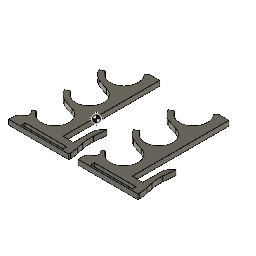
lokaverkefni_lappir_final (Autodesk Fusion 360 design; units mm, degrees)
Autodesk Fusion 360 part; units mm, degrees
sketch "Sketch1" plane through (0, 0, 0) normal (0, 0, 1) x (1, 0, 0)
  line L0 (34.445, 101.1531) -> (37.0871, 100)
  arc A0 (15.1934, 27.8106) -> (21.2794, 18.3659) centre (60, 50) ccw
  arc A1 (24.2675, 32.0225) -> (70.2683, 88.6596) centre (60, 50) ccw
  arc A2 (34.445, 101.1531) -> (70.2683, 88.6596) centre (134.445, 330.2819) ccw
  line L1 (50.2426, 114.2585) -> (49.0508, 111.5277)
  arc A3 (10.6816, 125.6547) -> (38.9202, 99.2) centre (60, 150) ccw
  arc A4 (24.2808, 131.9962) -> (70.2683, 188.6596) centre (60, 150) ccw
  arc A5 (36.6337, 200.2103) -> (70.2683, 188.6596) centre (134.445, 430.2819) ccw
  line L2 (88.2384, 278.3301) -> (95.3094, 285.4012)
  line L3 (60, 250) -> (120.6972, 250) construction
  arc A6 (24.2808, 231.9962) -> (88.2384, 278.3301) centre (60, 250) ccw
  arc A7 (10.6816, 225.6547) -> (36.6337, 200.2103) centre (60, 250) ccw
  line L4 (22.7381, 243.2768) -> (36.5507, 243.2768) construction
  line L5 (15.1934, 27.8106) -> (24.2675, 32.0225)
  line L6 (10.6816, 125.6547) -> (24.2808, 131.9962)
  line L7 (10.6816, 225.6547) -> (22.7381, 231.2768)
  line L8 (22.7381, 231.2768) -> (24.2808, 231.9962)
  line L9 (19.271, 3.8476) -> (10.7481, -2.1202)
  line L10 (22.2568, 7.1468) -> (4.2808, 7.1468) construction
  line L11 (8.9321, -3.3918) -> (9.2648, -3.3918) construction
  line L12 (132.7141, 248.2311) -> (132.6969, 250.0757)
  line L13 (7.8236, -5.3117) -> (6.5405, -7.5341)
  line L14 (8.9321, -3.3918) -> (9.2648, -3.3918) construction
  line L15 (168.0417, 91.0528) -> (216.7808, 91.0528) construction
  arc A8 (19.271, 3.8476) -> (21.2794, 18.3659) centre (13.5353, 12.0391) ccw
  arc A9 (10.7481, -2.1202) -> (7.8236, -5.3117) centre (16.4838, -10.3117) ccw
  arc A10 (6.5405, -7.5341) -> (5.2029, -12.3246) centre (15.2007, -12.5341) ccw
  line L16 (179.1661, -24.8465) -> (179.1661, -23.5067)
  line L17 (5.2029, -12.3246) -> (4.9961, -22.1946)
  line L18 (17.1671, -29.5067) -> (179.1661, -29.5067)
  line L19 (179.1661, -29.5067) -> (179.1661, -23.5067)
  line L20 (98.1666, -29.5067) -> (98.1666, -24.5067)
  line L21 (98.1666, -24.5067) -> (38.1666, -24.5067)
  line L22 (98.1666, -24.5067) -> (158.1666, -24.5067)
  line L23 (126.3128, 6.8881) -> (126.3128, 286.8881)
  line L24 (95.3094, 285.4012) -> (96.7963, 286.8881)
  line L25 (126.3128, 286.8881) -> (96.7963, 286.8881)
  line L26 (126.3128, 6.8881) -> (156.3128, 6.8881)
  line L27 (156.3128, 6.8881) -> (156.3128, 60.2423)
  line L28 (4.9412, -27.4331) -> (4.9412, -29.5067)
  line L29 (17.1671, -29.5067) -> (4.9412, -29.5067)
  arc A11 (4.9961, -22.1946) -> (4.9412, -27.4331) centre (254.9412, -27.4331) ccw
  line L30 (163.3423, 77.2129) -> (173.2834, 87.154)
  line L31 (156.3128, 70.1834) -> (180.3128, 70.1834) construction
  line L32 (173.2834, 87.154) -> (170.0976, 50.7401)
  line L33 (173.2834, 87.154) -> (226.6167, 87.154) construction
  line L34 (179.1661, -24.8465) -> (179.1661, -24.8301)
  line L35 (176.5391, -1.1543) -> (172.3137, 17.6514)
  arc A12 (170.0976, 50.7401) -> (172.3137, 17.6514) centre (277.6866, 41.3272) ccw
  arc A13 (179.1661, -24.8301) -> (176.5391, -1.1543) centre (71.1661, -24.8301) ccw
  arc A14 (163.3423, 77.2129) -> (156.3128, 60.2423) centre (180.3128, 60.2423) ccw
  line L36 (38.1666, -24.5067) -> (38.1666, -14.5067)
  line L37 (38.1666, -14.5067) -> (158.1666, -14.5067)
  line L38 (158.1666, -14.5067) -> (158.1666, -24.5067)
  point P0 (6.4321, -7.7219)
  point P1 (157.8394, 81.2593)
  point P2 (162.8123, 31.2811)
  point P3 (156.3128, 81.8881)
  point P4 (168.6351, 34.0236)
  point P5 (179.1661, -12.8465)
  dimension "d10" = 80
  dimension "d11" = 100
  dimension "d12" = 80
  dimension "d13" = 100
  dimension "d16" = 100
  dimension "d19" = 80
  dimension "d21" = 250
  dimension "d22" = 250
  dimension "d23" = 45
  dimension "d24" = 50
  dimension "d33" = 12
  dimension "d43" = 12
  dimension "d44" = 35
  dimension "d65" = 120
  dimension "d66" = 5
  dimension "d71" = 14.1421
  dimension "d74" = 60
  dimension "d79" = 10
  dimension "d80" = 10
  dimension "d81" = 10
  dimension "d92" = 6
  dimension "d93" = 5
  dimension "d94" = 60
  dimension "d95" = 60
  dimension "d230" = 280
  dimension "d233" = 30
  dimension "d234" = 75
  dimension "d238" = 250
  dimension "d239" = 24
  dimension "d240" = 45
  dimension "d241" = 95
  dimension "d242" = 53.3333
  dimension "d243" = 12
  dimension "d244" = 108
  dimension "d245" = 24
  dimension "d246" = 10
  dimension "d247" = 90
  dimension "d248" = 120
  dimension "d249" = 10
  constraint concentric A0 A1
  constraint concentric A6 A7
  constraint coincident L0.end A3
  constraint coincident L0 A3.end
  constraint tangent L0 A2
  constraint tangent A1 A2
  constraint coincident L1.end A4
  constraint tangent A4 A5
  constraint horizontal L3
  constraint coincident L3.start A6.centre
  constraint horizontal L4
  constraint horizontal L10
  constraint horizontal L11
  constraint horizontal L14
  constraint horizontal L15
  constraint tangent A0 A8
  constraint tangent L9 A8
  constraint coincident L11.start L9
  constraint coincident L11.start L13
  constraint tangent L9 A9
  constraint tangent L13 A9
  constraint coincident P0 L13
  constraint tangent L13 A10
  constraint coincident A9 L11.end
  constraint coincident A8 L10.start
  constraint vertical L16
  constraint tangent A10 L17
  constraint horizontal L18
  constraint vertical L19
  constraint midpoint L18 L20.start
  constraint perpendicular L18 L20
  constraint perpendicular L20 L21
  constraint perpendicular L20 L22
  constraint vertical L23
  constraint parallel L2 L24
  constraint horizontal L25
  constraint perpendicular L23 L26
  constraint perpendicular L26 L27
  constraint coincident P3 L27
  constraint vertical L28
  constraint horizontal L29
  constraint tangent L28 A11
  constraint tangent L17 A11
  constraint horizontal L31
  constraint horizontal L33
  constraint parallel L16 L34
  constraint coincident P4 L32
  constraint coincident P4 L35
  constraint tangent L32 A12
  constraint tangent L35 A12
  constraint coincident P5 L35
  constraint coincident P5 L34
  constraint tangent L35 A13
  constraint tangent L34 A13
  constraint equal A12 A13
  constraint coincident L31.start L30
  constraint coincident L27 L31.start
  constraint tangent L30 A14
  constraint tangent L27 A14
  constraint perpendicular L21 L36
  constraint perpendicular L37 L38
  measures "d10" diameter of A1
  measures "d11" distance of A0.centre A3.centre
  measures "d12" diameter of A4
  measures "d13" distance of A3.centre L3.start
  measures "d16" diameter of A0
  measures "d19" diameter of A6
  measures "d21" radius of A2
  measures "d22" radius of A5
  measures "d23" angle of L2 L3
  measures "d24" distance of L3.start L2.end
  measures "d33" distance of L3.end L12.end
  measures "d43" distance of L4.start L7.end
  measures "d44" angle of L9 L10
  measures "d65" angle of L13 L14
  measures "d66" distance of L11.start P0
  measures "d71" distance of P1 L15.start
  measures "d74" distance of L15.start P2
  measures "d79" radius of A8
  measures "d80" radius of A9
  measures "d81" radius of A10
  measures "d92" distance of L16.end L18.end
  measures "d93" distance of L20.start L20.end
  measures "d94" distance of L20.end L21.end
  measures "d95" distance of L20.end L22.end
  measures "d230" distance of L23.start L23.end
  measures "d233" distance of L23.start L26.end
  measures "d234" distance of L26.end P3
  measures "d238" radius of A11
  measures "d239" distance of L31.start L30.end
  measures "d240" angle of L30 L31
  measures "d241" angle of L32 L33
  measures "d242" distance of L30.end P4
  measures "d243" distance of L16.start P5
  measures "d244" radius of A12
  measures "d245" radius of A14
  measures "d246" distance of L21.end L36.end
  measures "d247" angle of L36 L37
  measures "d248" distance of L36.end L37.end
  measures "d249" distance of L37.end L22.end
extrude "Extrude1" add sketch "Sketch1" along normal blind 12 contours A0 A1 A2 A3 A4 A5 L2 A6 A7 L5 L6 L7 L8 L9 L13 A8 A9 A10 L16 L17 L18 L19 L23 L24 L25 L26 L27 L28 L29 A11 L30 L32 L34 L35 A12 A13 A14 makes body 1
copy_body "CopyPasteBodies1" bodies 1 makes body 2
move_body "Move1" bodies 2 to x (1, 0, 0) y (0, 1, 0) z (0, 0, 1) at (0, 0, 200)
ref_plane "WorkPlane1" through (98.1666, -24.5067, 6) normal (0, 1, 0) x (-1, 0, 0)
sketch "Sketch2" plane through (0, -24.5067, 0) normal (0, 1, 0) x (1, 0, 0)
  line L0 (0, 0) -> (120, 0)
  line L1 (120, 0) -> (120, -174)
  line L2 (120, -174) -> (0, -174)
  line L3 (0, -174) -> (0, 0)
  dimension "d103" = 120
  dimension "d104" = 174
  constraint horizontal L0
  constraint vertical L1
  constraint horizontal L2
  constraint vertical L3
  constraint coincident L0.start L3.end
  measures "d103" distance of L0.start L0.end
  measures "d104" distance of L0.start L2.end
extrude "Extrude2" add sketch "Sketch2" along normal blind 10 separate body makes body 3
sketch "Sketch3" plane through (0, -14.5067, 0) normal (0, 1, 0) x (-1, 0, 0)
  line L0 (0, 174) -> (-120, 174)
  line L1 (-120, 174) -> (-120, 0)
  line L2 (-120, 0) -> (0, 0)
  line L3 (0, 0) -> (0, 174)
  line L4 (-120, 0) -> (0, 0)
  line L5 (0, 0) -> (0, 17)
  line L6 (0, 17) -> (-120, 17)
  line L7 (-120, 17) -> (-120, 0)
  line L8 (0, 174) -> (-120, 174)
  line L9 (-120, 174) -> (-120, 157)
  line L10 (-120, 157) -> (0, 157)
  line L11 (0, 157) -> (0, 174)
  dimension "d107" = 120
  dimension "d108" = 17
  dimension "d109" = 120
  dimension "d110" = 17
  constraint horizontal L4
  constraint vertical L5
  constraint horizontal L6
  constraint vertical L7
  constraint coincident L1.end L2.start
  constraint horizontal L8
  constraint vertical L9
  constraint horizontal L10
  constraint vertical L11
  constraint coincident L0.start L3.end
  measures "d107" distance of L1.end L2.end
  measures "d108" distance of L1.end L6.end
  measures "d109" distance of L0.start L0.end
  measures "d110" distance of L0.start L10.end
extrude "Extrude3" cut sketch "Sketch3" against normal blind 4 contours L0 L1 L3 L8 L9 L10 L11 | L1 L2 L3 L4 L5 L6 L7 bodies 3
fillet "Fillet1" radius 6 2 edges at (120, -21.5067, 0) (0, -21.5067, 0) on bodies 3
fillet "Fillet2" radius 6 2 edges at (120, -21.5067, 174) (0, -21.5067, 174) on bodies 3
move_body "Move2" bodies 3 to x (1, 0, 0) y (0, 1, 0) z (0, 0, 1) at (0, 0, 32.3)
move_body "Move3" bodies 3 to x (1, 0, 0) y (0, 1, 0) z (0, 0, 1) at (36.8, 0, 0)
move_body "Move4" bodies 1 to x (1, 0, 0) y (0, 1, 0) z (0, 0, 1) at (0, 0, 40)
ref_plane "WorkPlane2" through (139.2808, 0, 206) normal (0, 1, 0) x (-1, 0, 0)
sketch "Sketch4" plane through (0, 0, 0) normal (0, 1, 0) x (1, 0, 0)
  line L0 (-0.6997, 0) -> (11.3003, 0)
  line L1 (11.3003, 0) -> (11.3003, 250)
  line L2 (11.3003, 250) -> (-0.6997, 250)
  line L3 (-0.6997, 250) -> (-0.6997, 0)
  dimension "d119" = 12
  dimension "d120" = 250
  constraint horizontal L0
  constraint vertical L1
  constraint horizontal L2
  constraint vertical L3
  measures "d119" distance of L0.start L0.end
  measures "d120" distance of L0.start L2.end
extrude "Extrude4" add sketch "Sketch4" along normal blind 150 separate body makes body 4
move_body "Move5" bodies 4 to x (1, 0, 0) y (0, 1, 0) z (0, 0, 1) at (130, 0, 230)
move_body "Move6" bodies 4 to x (1, 0, 0) y (0, 1, 0) z (0, 0, 1) at (0, 0, 25)
sketch "Sketch5" plane through (141.3003, 0, 0) normal (1, 0, 0) x (0, 1, 0)
  line L0 (0, 255) -> (0, 5)
  line L1 (0, 5) -> (150, 5)
  line L2 (150, 5) -> (150, 255)
  line L3 (150, 255) -> (0, 255)
  circle A0 centre (75, 225) radius 9
  dimension "d128" = 18
  measures "d128" diameter of A0
extrude "Extrude5" cut sketch "Sketch5" against normal blind 12 contours A0 bodies 4
fillet "Fillet3" radius 12 4 edges at (135.3003, 150, 5) (135.3003, 0, 5) (135.3003, 150, 255) (135.3003, 0, 255) on bodies 4
sketch "Sketch6" plane through (141.3003, 0, 0) normal (1, 0, 0) x (0, 1, 0)
  arc A0 (12, 255) -> (0, 243) centre (12, 243) ccw
  line L0 (0, 243) -> (0, 17)
  arc A1 (0, 17) -> (12, 5) centre (12, 17) ccw
  line L1 (12, 5) -> (138, 5)
  arc A2 (138, 5) -> (150, 17) centre (138, 17) ccw
  line L2 (150, 17) -> (150, 243)
  arc A3 (150, 243) -> (138, 255) centre (138, 243) ccw
  line L3 (138, 255) -> (12, 255)
  circle A4 centre (75, 225) radius 9
  line L4 (75, 10) -> (25, 10)
  line L5 (5, 30) -> (5, 230)
  line L6 (25, 250) -> (125, 250)
  line L7 (145, 230) -> (145, 30)
  line L8 (125, 10) -> (75, 10)
  arc A5 (5, 30) -> (25, 10) centre (25, 30) ccw
  arc A6 (25, 250) -> (5, 230) centre (25, 230) ccw
  arc A7 (145, 230) -> (125, 250) centre (125, 230) ccw
  arc A8 (125, 10) -> (145, 30) centre (125, 30) ccw
  line L9 (75, 10) -> (180, 10) construction
  line L10 (5, 80) -> (105, 80) construction
  line L11 (145, 80) -> (245, 80) construction
  line L12 (75, 150) -> (175, 150) construction
  line L13 (75, 150) -> (175, 150) construction
  line L14 (22, 19.1218) -> (122.3301, 19.1218)
  line L15 (134.3301, 31.1218) -> (134.3301, 225)
  line L16 (122.3301, 237) -> (22, 237)
  line L17 (10, 225) -> (10, 31.1218)
  arc A9 (22, 237) -> (10, 225) centre (22, 225) ccw
  arc A10 (134.3301, 225) -> (122.3301, 237) centre (122.3301, 225) ccw
  arc A11 (122.3301, 19.1218) -> (134.3301, 31.1218) centre (122.3301, 31.1218) ccw
  arc A12 (10, 31.1218) -> (22, 19.1218) centre (22, 31.1218) ccw
  line L18 (72.1651, 19.1218) -> (72.1651, 44.1218)
  line L19 (56.25, 65) -> (93.75, 65)
  line L20 (56.25, 27.5) -> (93.75, 27.5)
  arc A13 (56.25, 65) -> (56.25, 27.5) centre (56.25, 46.25) ccw
  arc A14 (93.75, 27.5) -> (93.75, 65) centre (93.75, 46.25) ccw
  line L21 (75, 65) -> (75, 190)
  line L22 (75, 190) -> (100, 190)
  line L23 (75, 190) -> (50, 190)
  line L24 (75, 190) -> (75, 158.75)
  line L25 (75, 158.75) -> (120, 158.75)
  circle A15 centre (120, 158.75) radius 12.5
  circle A16 centre (100, 190) radius 12.5
  circle A17 centre (50, 190) radius 12.5
  line L26 (75, 158.75) -> (30, 158.75)
  circle A18 centre (30, 158.75) radius 12.5
  line L27 (75, 158.75) -> (75, 127.5)
  line L28 (75, 127.5) -> (75, 96.25)
  line L29 (75, 96.25) -> (75, 65)
  line L30 (75, 127.5) -> (120, 127.5)
  line L31 (120, 127.5) -> (30, 127.5)
  circle A19 centre (120, 127.5) radius 12.5
  circle A20 centre (30, 127.5) radius 12.5
  line L32 (75, 96.25) -> (100, 96.25)
  circle A21 centre (100, 96.25) radius 12.5
  line L33 (75, 96.25) -> (73.5596, 96.25)
  line L34 (73.5596, 96.25) -> (48.5596, 96.25)
  circle A22 centre (48.5596, 96.25) radius 12.5
  circle A23 centre (75, 143.125) radius 25
  circle A24 centre (75, 143.125) radius 18.75
  point P0 (5, 10)
  point P1 (5, 250)
  point P2 (145, 250)
  point P3 (145, 10)
  point P4 (134.3301, 19.1218)
  point P5 (10, 237)
  dimension "d138" = 70
  dimension "d139" = 240
  dimension "d143" = 140
  dimension "d144" = 240
  dimension "d145" = 70
  dimension "d146" = 20
  dimension "d191" = 12
  dimension "d194" = 25
  dimension "d196" = 37.5
  dimension "d197" = 37.5
  dimension "d198" = 37.5
  dimension "d199" = 37.5
  dimension "d200" = 125
  dimension "d201" = 25
  dimension "d202" = 25
  dimension "d203" = 31.25
  dimension "d204" = 45
  dimension "d205" = 25
  dimension "d206" = 25
  dimension "d207" = 25
  dimension "d208" = 45
  dimension "d209" = 25
  dimension "d210" = 31.25
  dimension "d211" = 31.25
  dimension "d212" = 31.25
  dimension "d213" = 45
  dimension "d214" = 90
  dimension "d215" = 25
  dimension "d216" = 25
  dimension "d217" = 25
  dimension "d219" = 25
  dimension "d220" = 25
  dimension "d221" = 25
  dimension "d224" = 50
  dimension "d225" = 37.5
  constraint perpendicular L1 L5
  constraint perpendicular L5 L6
  constraint perpendicular L6 L7
  constraint perpendicular L7 L8
  constraint coincident P0 L4
  constraint coincident P0 L5
  constraint tangent L4 A5
  constraint tangent L5 A5
  constraint coincident P1 L5
  constraint coincident P1 L6
  constraint tangent L5 A6
  constraint tangent L6 A6
  constraint equal A5 A6
  constraint coincident P2 L7
  constraint coincident P2 L6
  constraint tangent L7 A7
  constraint tangent L6 A7
  constraint equal A5 A7
  constraint coincident P3 L7
  constraint coincident P3 L8
  constraint tangent L7 A8
  constraint tangent L8 A8
  constraint equal A5 A8
  constraint horizontal L9
  constraint coincident L5 L10.start
  constraint horizontal L10
  constraint horizontal L11
  constraint coincident L7 L11.start
  constraint horizontal L12
  constraint horizontal L13
  constraint horizontal L14
  constraint vertical L15
  constraint horizontal L16
  constraint vertical L17
  constraint coincident P5 L17
  constraint coincident P5 L16
  constraint tangent L17 A9
  constraint tangent L16 A9
  constraint tangent L15 A10
  constraint tangent L16 A10
  constraint equal A9 A10
  constraint coincident P4 L14
  constraint coincident P4 L15
  constraint tangent L14 A11
  constraint tangent L15 A11
  constraint equal A9 A11
  constraint tangent L14 A12
  constraint tangent L17 A12
  constraint equal A9 A12
  constraint midpoint L14 L18.start
  constraint perpendicular L14 L18
  constraint horizontal L19
  constraint tangent L20 A13
  constraint perpendicular L18 L20
  constraint midpoint L19 L21.start
  constraint perpendicular L19 L21
  constraint perpendicular L21 L22
  constraint perpendicular L21 L23
  constraint perpendicular L13 L24
  constraint perpendicular L24 L25
  constraint coincident L25.end A15.centre
  constraint coincident L22.end A16.centre
  constraint coincident L23.end A17.centre
  constraint perpendicular L21 L26
  constraint coincident L26.end A18.centre
  constraint perpendicular L12 L27
  constraint perpendicular L12 L28
  constraint perpendicular L10 L29
  constraint perpendicular L28 L30
  constraint perpendicular L28 L31
  constraint coincident L30.end L31.start
  constraint coincident L31.end A20.centre
  constraint perpendicular L28 L32
  constraint coincident L32.end A21.centre
  constraint perpendicular L28 L33
  constraint perpendicular L28 L34
  constraint coincident L34.end A22.centre
  constraint midpoint L27 A23.centre
  constraint concentric A23 A24
  measures "d138" distance of L4.start P0
  measures "d139" distance of P0 P1
  measures "d143" distance of P1 P2
  measures "d144" distance of P2 P3
  measures "d145" distance of P3 L4.start
  measures "d146" radius of A5
  measures "d191" radius of A9
  measures "d194" distance of L18.start L18.end
  measures "d196" diameter of A14
  measures "d197" diameter of A13
  measures "d198" distance of L19.start L19.end
  measures "d199" distance of L20.start L20.end
  measures "d200" distance of L21.start L21.end
  measures "d201" distance of L21.end L22.end
  measures "d202" distance of L21.end L23.end
  measures "d203" distance of L21.end L24.end
  measures "d204" distance of L24.end L25.end
  measures "d205" diameter of A15
  measures "d206" diameter of A16
  measures "d207" diameter of A17
  measures "d208" distance of L24.end L26.end
  measures "d209" diameter of A18
  measures "d210" distance of L24.end L27.end
  measures "d211" distance of L27.end L28.end
  measures "d212" distance of L28.end L21.start
  measures "d213" distance of L27.end L30.end
  measures "d214" distance of L30.end L31.end
  measures "d215" diameter of A19
  measures "d216" diameter of A20
  measures "d217" distance of L28.end L32.end
  measures "d219" diameter of A21
  measures "d220" distance of L33.end L34.end
  measures "d221" diameter of A22
  measures "d224" diameter of A23
  measures "d225" diameter of A24
extrude "Extrude6" cut sketch "Sketch6" against normal blind 5 contours A4 | L4 L5 L6 L7 L8 A5 A6 A7 A8 | L14 L15 L16 L17 A9 A10 A11 A12 | L19 L20 A13 A14 | L21 L26 L27 L31 A24 | L21 L28 L30 L31 A24 | L21 L25 L27 L30 L31 A24 | L21 L28 L31 A24 | L21 L24 L26 A24 | L21 L24 L25 A24 | L21 L28 L30 L31 A23 A24 | L21 L28 L31 A23 A24 | L25 L30 L31 A23 A24 | L26 L31 A23 A24 | L21 L24 L26 A23 A24 | L21 L24 L25 A23 A24 | A15 | A16 | A17 | A18 | A19 | A20 | A21 | A22 bodies 4
copy_body "CopyPasteBodies2" bodies 4 makes body 5
move_body "Move7" bodies 5 to x (1, 0, 0) y (0, 1, 0) z (0, 0, 1) at (100, 0, 0)
extrude "Extrude7" cut sketch "Sketch6" against normal blind 6 contours L4 L5 L6 L7 L8 A5 A6 A7 A8 bodies 4
extrude "Extrude8" cut sketch "Sketch6" against normal blind 6 contours L4 L5 L6 L7 L8 A5 A6 A7 A8 | L19 L20 A13 A14 | L21 L28 L30 L31 A23 A24 | L21 L28 L31 A23 A24 | L25 L30 L31 A23 A24 | L26 L31 A23 A24 | L21 L24 L26 A23 A24 | L21 L24 L25 A23 A24 | A15 | A16 | A17 | A18 | A19 | A20 | A21 | A22 bodies 4
extrude "Extrude9" cut sketch "Sketch6" against normal blind 6 contours L19 L20 A13 A14 | L21 L28 L30 L31 A23 A24 | L21 L28 L31 A23 A24 | L25 L30 L31 A23 A24 | L26 L31 A23 A24 | L21 L24 L26 A23 A24 | L21 L24 L25 A23 A24 | A15 | A16 | A17 | A18 | A19 | A20 | A21 | A22 bodies 4
extrude "Extrude10" add sketch "Sketch1" along normal blind 12 separate body contours A0 A1 A2 A3 A4 A5 L2 A6 A7 L5 L6 L7 L8 L9 L13 A8 A9 A10 L16 L17 L18 L19 L23 L24 L25 L26 L27 L28 L29 A11 L30 L32 L34 L35 A12 A13 A14 makes body 6
move_body "Align1" bodies 2 to x (1, 0, 0) y (0, 1, 0) z (0, 0, 1) at (0, 0, -160)
move_body "Move8" bodies 2 to x (1, 0, 0) y (0, 1, 0) z (0, 0, 1) at (200, 0, 0)
extrude "Extrude11" add 2 faces at (117.5398, 114.3561, 40) (317.5398, 114.3561, 40) along direction (0, 0, -1) blind 3 on bodies 1 2 bodies 1 2
hidden bodies 3 4 5 6
equation "lengd_x = 150 mm"
equation "lengd_y = 250 mm"
equation "þykkt = 10 mm"
equation "bottle = 80 mm"
equation "d10 = bottle"
equation "d11 = lengd_x / 3 * 2"
equation "d12 = bottle"
equation "d13 = lengd_x / 3 * 2"
equation "d16 = bottle + þykkt * 2"
equation "d19 = bottle"
equation "d21 = lengd_y"
equation "d22 = lengd_y"
equation "d23 = 90 deg - 45 deg"
equation "d24 = bottle / 2 + þykkt"
equation "THICK = 12 mm"
equation "d33 = THICK"
equation "d43 = THICK"
equation "lengd_dx = lengd_x - 3 * þykkt"
equation "d66 = þykkt / 2"
equation "d71 = þykkt / cos(45 deg)"
equation "d74 = lengd_dx / 2"
equation "d79 = þykkt"
equation "d80 = þykkt"
equation "d81 = þykkt"
equation "d92 = THICK / 2"
equation "d93 = þykkt / 2"
equation "d94 = lengd_dx / 2"
equation "d95 = lengd_dx / 2"
equation "d99 = THICK"
equation "y_plata = 140 mm + THICK * 2 + þykkt"
equation "d103 = lengd_dx"
equation "d104 = y_plata"
equation "d105 = þykkt"
equation "d107 = lengd_dx"
equation "d108 = THICK + þykkt / 2"
equation "d109 = lengd_dx"
equation "d110 = THICK + þykkt / 2"
equation "d111 = THICK / 2 - þykkt"
equation "d114 = THICK / 2"
equation "d116 = THICK / 2"
equation "skurdarbretti = 250 mm"
equation "d119 = THICK"
equation "d120 = skurdarbretti"
equation "d121 = lengd_x"
equation "d128 = THICK * 1.5"
equation "d129 = -THICK"
equation "d132 = THICK"
equation "endar_bretti = skurdarbretti * 0.02"
equation "kassi_skurbretti = skurdarbretti / 2 - endar_bretti * 4"
equation "d138 = lengd_x / 2 - endar_bretti"
equation "d143 = lengd_x - 2 * endar_bretti"
equation "d144 = skurdarbretti - 2 * endar_bretti"
equation "d145 = lengd_x / 2 - endar_bretti"
equation "d168 = -endar_bretti"
equation "skot_þvermal = 25 mm"
equation "d191 = THICK"
equation "d192 = -THICK / 2"
equation "d194 = skot_þvermal"
equation "d196 = skot_þvermal * 1.5"
equation "d197 = skot_þvermal * 1.5"
equation "d198 = skot_þvermal * 1.5"
equation "d199 = skot_þvermal * 1.5"
equation "d200 = skurdarbretti / 2"
equation "d201 = skot_þvermal"
equation "d202 = skot_þvermal"
equation "d203 = skurdarbretti / 2 * 0.25"
equation "d204 = skot_þvermal * 1.8"
equation "d205 = skot_þvermal"
equation "d206 = skot_þvermal"
equation "d207 = skot_þvermal"
equation "d208 = skot_þvermal * 1.8"
equation "d209 = skot_þvermal"
equation "d210 = skurdarbretti / 2 * 0.25"
equation "d211 = skurdarbretti / 2 * 0.25"
equation "d212 = skurdarbretti / 2 * 0.25"
equation "d213 = skot_þvermal * 1.8"
equation "d214 = skot_þvermal * 2 * 1.8"
equation "d215 = skot_þvermal"
equation "d216 = skot_þvermal"
equation "d217 = skot_þvermal"
equation "d219 = skot_þvermal"
equation "d220 = skot_þvermal"
equation "d221 = skot_þvermal"
equation "d224 = skot_þvermal * 2"
equation "d225 = skot_þvermal * 1.5"
equation "d226 = -THICK / 2"
equation "d228 = -THICK / 2"
equation "d230 = lengd_y + þykkt * 3"
equation "d233 = THICK * 2 + þykkt / 2 + 1 mm"
equation "d234 = lengd_x / 2"
equation "d238 = lengd_y"
equation "d239 = THICK * 2"
equation "d242 = bottle / 1.5"
equation "d243 = THICK"
equation "d244 = THICK * 9"
equation "d245 = THICK * 2"
equation "d246 = þykkt"
equation "d248 = lengd_dx"
equation "d249 = þykkt"
equation "d250 = THICK"
